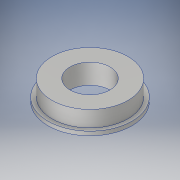
# Autodesk Inventor part: F6800_2019
Saved by Autodesk Inventor 2019.4 (Build 234330000, 330)
## iProperties
Created: 2020-02-07
Part Number: F6800_2019
Material: Aluminum 6061
Document SubType Name: Modeling
Designer: Paul Lefeuvre
Density: 2.7 g/cm^3
Appearance: Aluminum - Flat
Author: Paul Lefeuvre
Autodesk Inventor part; units mm, degrees
ref_plane "YZ Plane" through (0, 0, 0) normal (1, 0, 0) x (0, 1, 0)
ref_plane "XZ Plane" through (0, 0, 0) normal (0, 1, 0) x (-1, 0, 0)
ref_plane "XY Plane" through (0, 0, 0) normal (0, 0, 1) x (1, 0, 0)
sketch "Sketch1" plane through (0, 0, 0) normal (0, 0, 1) x (1, 0, 0)
  line L0 (0, 0) -> (0, 7.3794)
  line L1 (5, 0) -> (10.5, 0)
  line L2 (10.5, 0) -> (10.5, 1)
  line L3 (5, 5) -> (9.5, 5)
  line L4 (9.5, 5) -> (9.5, 1)
  line L5 (9.5, 1) -> (10.5, 1)
  line L6 (5, 5) -> (5, 0)
  dimension "d0" = 1
  dimension "d1" = 10.5
  dimension "d2" = 9.5
  dimension "d3" = 4
  dimension "d4" = 5
  constraints: 15 end point, 4 perpendicular, 2 horizontal, 1 point on line, 1 vertical
  measures "d0" distance of L1.end L2.end
  measures "d1" distance between parallel lines of L0 L2
  measures "d2" distance between parallel lines of L0 L4
  measures "d3" distance of L3.end L4.end
  measures "d4" distance between parallel lines of L0 L6
revolve "Revolution1" add sketch "Sketch1" angle 360 about axis through (0, 0, 0) along (0, 1, 0)
body "Solid1"
